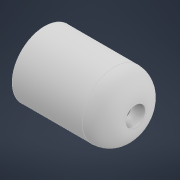
# Autodesk Inventor part: 12
Saved by Autodesk Inventor 2021.2 (Build 252289000, 289)
## iProperties
Created: 2023-09-07
Part Number: 12
Material: Типовые
Document SubType Name: Modeling
Designer: User
Density: 1 g/cm^3
Appearance: По умолчанию
Author: User
Autodesk Inventor part; units mm, degrees
ref_plane "YZ Plane" through (0, 0, 0) normal (1, 0, 0) x (0, 1, 0)
ref_plane "XZ Plane" through (0, 0, 0) normal (0, 1, 0) x (-1, 0, 0)
ref_plane "XY Plane" through (0, 0, 0) normal (0, 0, 1) x (1, 0, 0)
sketch "Блок1" plane through (0, 0, 0) normal (0, 0, 1) x (1, 0, 0)
  line L0 (-20.8941, 6.9119) -> (-9.8941, 6.9119)
  line L1 (-8.8941, 8.4119) -> (-6.8941, 8.4119)
  point P0 (-11.6441, 7.6619)
sketch "Эскиз1" plane through (0, 0, 0) normal (0, 0, 1) x (1, 0, 0)
  line L0 (0.0239, 0.0663) -> (10.8239, 0.0663)
  line L1 (14.0239, 3.2663) -> (14.0239, 3.5663)
  arc A0 (10.8239, 0.0663) -> (14.0239, 3.2663) centre (10.8239, 3.2663) ccw
  line L2 (0.0239, 0.0663) -> (0.0239, 2.0663)
  line L3 (12.0239, 3.0663) -> (12.0239, 3.5663)
  arc A1 (11.0239, 2.0663) -> (12.0239, 3.0663) centre (11.0239, 3.0663) ccw
  line L4 (14.0239, 3.5663) -> (14.0239, 5.0663)
  line L5 (0.0239, 5.0663) -> (7.906, 5.0663)
  line L6 (0.0239, 2.0663) -> (11.0239, 2.0663)
  line L7 (12.0239, 3.5663) -> (14.0239, 3.5663)
  point P0 (0, 0)
  point P1 (14.0239, 0.0663)
  point P2 (11.0239, 2.0663)
  dimension "d8" = 2
  dimension "d15" = 3.2
  dimension "d18" = 5
  dimension "d19" = 10.8
  constraints: 12 end point, 4 point on circle, 4 tangent, 2 centre point, 2 horizontal, 2 perpendicular, 2 point on line, 1 vertical, 5 other
  measures "d8" distance of L0.start L2.end
  measures "d15" radius of A0
  measures "d18" distance between parallel lines of L0 L5
  measures "d19" distance of L0.start L0.end
revolve "Вращение1" add sketch "Эскиз1" angle 360 about axis through (0.0239, 5.0663, 0) along (1, 0, 0)
